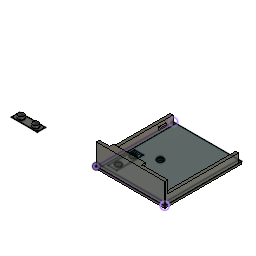
POWERDIAG_OBI_CASE_2 (Autodesk Fusion 360 design; units mm, degrees)
part number: 2026-08-31-23-20-56-590
Autodesk Fusion 360 part; units mm, degrees
note: some values were not read from the file. Set by a fixed rule: which face or edge a step refers to.
sketch "Sketch1" plane through (0, 0, 0) normal (0, 0, 1) x (1, 0, 0)
  line L0 (0, 0) -> (46.5, 0)
  line L1 (46.5, 0) -> (46.5, 52.2)
  line L2 (46.5, 52.2) -> (0, 52.2)
  line L3 (0, 52.2) -> (0, 0)
  line L4 (46.5, 2) -> (0, 2)
  line L5 (44.5, 52.2) -> (44.5, 2)
  line L6 (2, 52.2) -> (2, 2)
  circle A0 centre (6.5, 8.5) radius 2
  circle A1 centre (6.5, 18.5) radius 2
  line L7 (3.5, 22.5) -> (9.5, 22.5)
  line L8 (9.5, 22.5) -> (9.5, 4.5)
  line L9 (9.5, 4.5) -> (3.5, 4.5)
  line L10 (3.5, 4.5) -> (3.5, 22.5)
  circle A2 centre (18, 25.5) radius 2
  dimension "d1" = 46.5
  dimension "d2" = 52.2
  dimension "d3" = 2
  dimension "d4" = 2
  dimension "d5" = 2
  dimension "d55" = 6.5
  dimension "d56" = 6.5
  dimension "d57" = 4
  dimension "d58" = 4
  dimension "d59" = 6.5
  dimension "d60" = 10
  dimension "d61" = 4
  dimension "d62" = 4
  dimension "d63" = 3
  dimension "d64" = 3
  dimension "d70" = 23.5
  dimension "d72" = 18
  dimension "d73" = 4
  constraint horizontal L0
  constraint vertical L1
  constraint horizontal L2
  constraint vertical L3
  constraint coincident L0.start L3.end
  constraint coincident L1 L4.start
  constraint coincident L3 L4.end
  constraint perpendicular L3 L4
  constraint coincident L2 L5.start
  constraint coincident L4 L5.end
  constraint perpendicular L4 L5
  constraint coincident L2 L6.start
  constraint coincident L4 L6.end
  constraint perpendicular L4 L6
  constraint horizontal L7
  constraint vertical L8
  constraint horizontal L9
  constraint vertical L10
  measures "d1" distance of L0.start L0.end
  measures "d2" distance of L0.end L1.end
  measures "d3" distance of L0 L4
  measures "d4" distance of L3 L6
  measures "d5" distance of L1 L5
  measures "d55" distance of L3 A0.centre
  measures "d56" distance of L4 A0.centre
  measures "d57" diameter of A0
  measures "d58" diameter of A1
  measures "d59" distance of L3 A1.centre
  measures "d60" distance of A0.centre A1.centre
  measures "d61" distance of A0.centre L9
  measures "d62" distance of A1.centre L7
  measures "d63" distance of A1.centre L8
  measures "d64" distance of A1.centre L10
  measures "d70" distance of L4 A2.centre
  measures "d72" distance of L3 A2.centre
  measures "d73" diameter of A2
extrude "Extrude1" add sketch "Sketch1" against normal blind 2 contours L0 L1 L3 L4 | L2 L3 L4 L6 | L1 L2 L4 L5 | L2 L4 L5 L6 | A0 | A1 | L7 L8 L9 L10 | A2 makes body 1
extrude "Extrude2" add sketch "Sketch1" along normal blind 6 contours L2 L3 L4 L6 | L1 L2 L4 L5 bodies 1
extrude "Extrude3" add sketch "Sketch1" along normal blind 14.3 contours L0 L1 L3 L4 bodies 1
sketch "Sketch2" plane through (0, 0, 0) normal (-1, 0, 0) x (0, -1, 0)
  line L0 (-52.2, 6) -> (-52.2, -2)
  line L1 (-52.2, -2) -> (0, -2)
  line L2 (0, -2) -> (0, 14.3)
  line L3 (0, 14.3) -> (-2, 14.3)
  line L4 (-2, 14.3) -> (-2, 6)
  line L5 (-2, 6) -> (-52.2, 6)
  line L6 (-52.2, 6) -> (-50.2, 6)
  line L7 (-50.2, 6) -> (-50.2, 0)
  line L8 (-50.2, 0) -> (-52.2, 0)
  line L9 (-52.2, 0) -> (-52.2, 6)
  line L10 (-52.2, 0) -> (0, 0)
  dimension "d12" = 2
  constraint horizontal L6
  constraint vertical L7
  constraint horizontal L8
  constraint vertical L9
  constraint coincident L0.start L5.end
  constraint collinear L8 L10
  measures "d12" distance of L0.start L6.end
extrude "Extrude4" cut sketch "Sketch2" against normal up to surface (46.5 mm away) contours L0 L5 L6 L7 L8 L9 L10 bodies 1
sketch "Sketch3" plane through (44.5, 0, 0) normal (-1, 0, 0) x (0, -1, 0)
  line L0 (-50.2, 6) -> (-50.2, 0)
  line L1 (-50.2, 0) -> (-2, 0)
  line L2 (-2, 0) -> (-2, 6)
  line L3 (-2, 6) -> (-50.2, 6)
  line L4 (-45.2, 4) -> (-40.2, 4)
  line L5 (-40.2, 4) -> (-40.2, 2)
  line L6 (-40.2, 2) -> (-45.2, 2)
  line L7 (-45.2, 2) -> (-45.2, 4)
  dimension "d15" = 2
  dimension "d16" = 5
  dimension "d17" = 2
  dimension "d18" = 5
  constraint horizontal L4
  constraint vertical L5
  constraint horizontal L6
  constraint vertical L7
  measures "d15" distance of L3 L4
  measures "d16" distance of L5 L7
  measures "d17" distance of L4 L6
  measures "d18" distance of L0 L7
extrude "Extrude5" add sketch "Sketch3" along normal blind 0.8 contours L4 L5 L6 L7 bodies 1
pattern_linear "R-Pattern1" count 2 spacing 30 along (0, -1, 0) of "Extrude5"
ref_plane "WorkPlane1" through (23.25, 27.1, 3) normal (-1, 0, 0) x (0, -1, 0)
mirror "Mirror1" about plane through (23.25, 27.1, 3) normal (-1, 0, 0) of "Extrude5", "R-Pattern1"
chamfer "Chamfer1" distance 0.6 angle 45 4 faces at (43.7, 43.5333, 3.3333) (43.7, 13.5333, 3.3333) (2.8, 43.5333, 3.3333) (2.8, 13.5333, 3.3333) on bodies 1
sketch "Sketch4" plane through (0, 2, 0) normal (0, 1, 0) x (-1, 0, 0)
  line L0 (-46.5, 6) -> (-44.5, 6)
  line L1 (-44.5, 6) -> (-44.5, 0)
  line L2 (-44.5, 0) -> (-2, 0)
  line L3 (-2, 0) -> (-2, 6)
  line L4 (-2, 6) -> (0, 6)
  line L5 (0, 6) -> (0, 14.3)
  line L6 (0, 14.3) -> (-46.5, 14.3)
  line L7 (-46.5, 14.3) -> (-46.5, 6)
  line L8 (-7, 14.3) -> (-29, 14.3)
  line L9 (-29, 14.3) -> (-29, 11.7)
  line L10 (-29, 11.7) -> (-7, 11.7)
  line L11 (-7, 11.7) -> (-7, 14.3)
  dimension "d28" = 2.6
  dimension "d29" = 22
  dimension "d30" = 7
  constraint horizontal L8
  constraint vertical L9
  constraint horizontal L10
  constraint vertical L11
  constraint coincident L6 L8.start
  measures "d28" distance of L8.end L9.end
  measures "d29" distance of L9.end L10.end
  measures "d30" distance of L5 L11
extrude "Extrude6" add sketch "Sketch4" along normal blind 2.5 contours L6 L8 L9 L10 L11 bodies 1
extrude "Extrude8" cut sketch "Sketch1" against normal through all contours A2 bodies 1
chamfer "Chamfer2" distance 0.4 angle 45 3 edges at (46.5, 26.1, -2) (23.25, 0, -2) (0, 26.1, -2) on bodies 1
chamfer "Chamfer2" distance 0.3 angle 45 2 edges at (46.5, 0, 6.15) (0, 0, 6.15) on bodies 1
chamfer "Chamfer2" distance 2 angle 45 1 edges at (18, 4.5, 11.7) on bodies 1
extrude "Extrude9" cut sketch "Sketch1" against normal blind 1 contours L7 L8 L9 L10 bodies 1
extrude "Extrude10" cut sketch "Sketch1" against normal up to surface (2 mm away) contours A0 | A1 bodies 1
chamfer "Chamfer3" distance 0.5 angle 45 2 edges at (4.6353, 17.7768, -2) (4.6353, 7.7768, -2) on bodies 1
sketch "Sketch5" plane through (0, 0, 0) normal (0, 0, 1) x (1, 0, 0)
  line L0 (-57.6, 5.6) -> (-40, 5.6)
  line L1 (-40, 5.6) -> (-40, 0)
  line L2 (-40, 0) -> (-57.6, 0)
  line L3 (-57.6, 0) -> (-57.6, 5.6)
  line L4 (0, 52.2) -> (0, 0)
  line L5 (0, 0) -> (46.5, 0)
  circle A0 centre (-53.8, 2.8) radius 1.9
  circle A1 centre (-43.8, 2.8) radius 1.9
  dimension "d74" = 17.6
  dimension "d75" = 5.6
  dimension "d76" = 40
  dimension "d77" = 3.8
  dimension "d78" = 3.8
  dimension "d79" = 2.8
  dimension "d80" = 2.8
  dimension "d81" = 10
  dimension "d82" = 3.8
  constraint horizontal L0
  constraint vertical L1
  constraint horizontal L2
  constraint vertical L3
  constraint collinear L2 L5
  measures "d74" distance of L0.start L0.end
  measures "d75" distance of L0.end L1.end
  measures "d76" distance of L1 L4
  measures "d77" diameter of A1
  measures "d78" diameter of A0
  measures "d79" distance of L0 A0.centre
  measures "d80" distance of L0 A1.centre
  measures "d81" distance of A0.centre A1.centre
  measures "d82" distance of L3 A0.centre
extrude "Extrude11" add sketch "Sketch5" along normal blind 2 separate body contours A0 | A1 makes body 2 at (-51.9024, 2.7053, 1.3333) makes body 3 at (-41.9024, 2.7053, 1.3333)
extrude "Extrude12" add sketch "Sketch5" along normal blind 0.2 bodies 2 3
fillet "Fillet1" radius 2 4 edges at (-57.6, 0, 0.1) (-57.6, 5.6, 0.1) (-40, 5.6, 0.1) (-40, 0, 0.1) on bodies 2
equation "d80 = d79"
